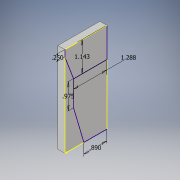
# Autodesk Inventor part: Suspension I
Saved by Autodesk Inventor 2018 (Build 220112000, 112)
## iProperties
Created: 2017-10-30
Part Number: Suspension I
Material: Generic
Document SubType Name: Modeling
Designer: Intel
Density: 1 g/cm^3
Appearance: Default
Author: Intel
Autodesk Inventor part; units mm, degrees
ref_plane "YZ Plane" through (0, 0, 0) normal (1, 0, 0) x (0, 1, 0)
ref_plane "XZ Plane" through (0, 0, 0) normal (0, 1, 0) x (-1, 0, 0)
ref_plane "XY Plane" through (0, 0, 0) normal (0, 0, 1) x (1, 0, 0)
sketch "Sketch1" plane through (0, 0, 0) normal (0, 1, 0) x (-1, 0, 0)
  line L0 (0, 1.6817) -> (6.731, 1.6817)
  line L1 (6.731, 1.6817) -> (6.731, -39.5171)
  line L2 (6.731, -39.5171) -> (0, -39.5171)
  line L3 (0, -39.5171) -> (0, 1.6817)
  point P0 (0, 0)
  dimension "d0" = 6.731
  dimension "d1" = 41.1988
  constraints: 8 end point, 2 parallel, 1 horizontal, 1 perpendicular
  measures "d0" distance of L1.end L2.end
  measures "d1" distance of L0.end L1.end
extrude "Extrusion1" add sketch "Sketch1" along normal blind 88.1888
sketch "Sketch2" plane through (0, 0, 1.6817) normal (1, 0, 0) x (0, 0, -1)
  line L0 (0, 88.1888) -> (41.1988, 88.1888) projected
  line L1 (41.1988, 88.1888) -> (41.1988, 59.1566)
  line L2 (41.1988, 0) -> (41.1988, 88.1888) projected
  line L3 (41.1988, 59.1566) -> (8.4836, 59.1566)
  line L4 (8.4836, 59.1566) -> (8.4836, 34.3916)
  line L5 (41.1988, 0) -> (0, 0) projected
  line L6 (41.1988, 0) -> (18.5928, 0)
  line L7 (18.5928, 0) -> (8.4836, 34.3916)
  line L8 (0, 0) -> (0, 88.1888) projected
  line L9 (0, 88.1888) -> (0, 81.8388)
  line L10 (8.4836, 59.1566) -> (0, 81.8388)
  point P0 (1.6817, 0)
  dimension "d4" = 29.0322
  dimension "d5" = 32.7152
  dimension "d6" = 24.765
  dimension "d7" = 22.606
  dimension "d8" = 6.35
  constraints: 14 end point, 3 point on line, 1 horizontal, 1 vertical
  measures "d4" distance of L0.end L1.end
  measures "d5" distance of L1.end L3.end
  measures "d6" distance of L3.end L4.end
  measures "d7" distance of L2.start L6.end
  measures "d8" distance of L0.start L9.end
body "Solid1"
